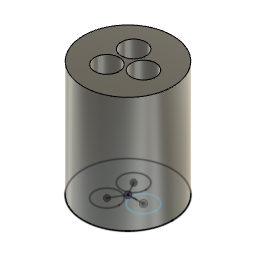
3 motor holder v1 (Autodesk Fusion 360 design; units mm, degrees)
Autodesk Fusion 360 part; units mm, degrees
sketch "Sketch1" plane through (0, 0, 0) normal (0, 0, 1) x (1, 0, 0)
  circle A0 centre (0, 0) radius 34.5
  line L0 (0, 0) -> (12, 0)
  line L1 (0, 0) -> (-6, 10.3923)
  line L2 (0, 0) -> (12, 0) construction
  line L3 (0, 0) -> (-6, -10.3923)
  line L4 (0, 0) -> (12, 0) construction
  circle A1 centre (-6, 10.3923) radius 9.5
  circle A2 centre (12, 0) radius 9.5
  circle A3 centre (-6, -10.3923) radius 9.5
  dimension "d1" = 69
  dimension "d2" = 12
  dimension "d3" = 12
  dimension "d4" = 120
  dimension "d5" = 120
  dimension "d6" = 12
  dimension "d7" = 19
  dimension "d8" = 19
  dimension "d9" = 19
  constraint coincident A0.centre L0.start
  constraint horizontal L0
  constraint horizontal L2
  constraint horizontal L4
  constraint coincident L1.end A1.centre
  constraint coincident L0.end L2.end
  constraint coincident L3.end A3.centre
  measures "d1" diameter of A0
  measures "d2" distance of A0.centre L0.end
  measures "d3" distance of A0.centre L1.end
  measures "d4" angle of L1 L2
  measures "d5" angle of L3 L4
  measures "d6" distance of A0.centre L3.end
  measures "d7" diameter of A1
  measures "d8" diameter of A2
  measures "d9" diameter of A3
extrude "Extrude1" add sketch "Sketch1" along normal blind 100
extrude "Extrude2" add sketch "Sketch1" along normal blind 20 contours A1 | A2 | A3
extrude "Extrude3" cut 1 faces at (10.3664, 17.9552, 100) along direction (0, 0, -1) blind 30
extrude "Extrude4" add 1 faces at (10.3664, 17.9552, 70) along direction (0, 0, 1) blind 20
